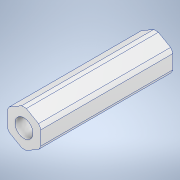
# Autodesk Inventor part: DriveShaft
Saved by Autodesk Inventor 2020 (Build 240168000, 168)
## iProperties
Created: 2019-06-24
Part Number: DriveShaft
Material: Aluminum 6061
Document SubType Name: Modeling
Designer: Connor
Density: 2.7 g/cm^3
Appearance: Smooth - Black
Mass: 13.5849 g
Surface Area: 33.5142 cm^2
Volume: 5.03143 cm^3
Author: Connor
Autodesk Inventor part; units mm, degrees
ref_plane "YZ Plane" through (0, 0, 0) normal (1, 0, 0) x (0, 1, 0)
ref_plane "XZ Plane" through (0, 0, 0) normal (0, 1, 0) x (-1, 0, 0)
ref_plane "XY Plane" through (0, 0, 0) normal (0, 0, 1) x (1, 0, 0)
sketch "Sketch1" plane through (0, 0, 0) normal (0, 0, 1) x (1, 0, 0)
  line L0 (0, 7.3323) -> (6.35, 3.6662)
  line L1 (6.35, 3.6662) -> (6.35, -3.6662)
  line L2 (6.35, -3.6662) -> (0, -7.3323)
  line L3 (0, -7.3323) -> (-6.35, -3.6662)
  line L4 (-6.35, -3.6662) -> (-6.35, 3.6662)
  line L5 (-6.35, 3.6662) -> (0, 7.3323)
  circle A0 centre (0, 0) radius 6.875
  circle A1 centre (0, 0) radius 3.3734
  point P0 (-5.457, 4.1818)
  point P1 (-6.35, 2.635)
  point P2 (-6.35, -2.635)
  point P3 (-5.457, -4.1818)
  point P4 (-0.893, -6.8168)
  point P5 (0.893, -6.8168)
  point P6 (5.457, -4.1818)
  point P7 (6.35, -2.635)
  point P8 (6.35, 2.635)
  point P9 (5.457, 4.1818)
  point P10 (0.893, 6.8168)
  point P11 (-0.893, 6.8168)
  dimension "d0" = 12.7
  dimension "d1" = 13.75
  dimension "d2" = 6.7469
  constraints: 12 end point, 3 coincident, 2 centre point, 1 vertical alignment, 13 other
  measures "d0" distance between parallel lines of L1 L4
  measures "d1" diameter of A0
  measures "d2" diameter of A1
extrude "Extrusion1" add sketch "Sketch1" along normal blind 49.53 contours L0 A0 L1 L2 L3 L4 L5
body "Solid1"
